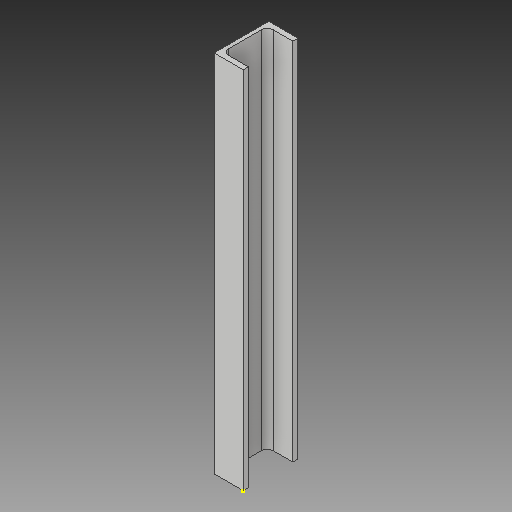
# Autodesk Inventor part: Channel2_CPY
Saved by Autodesk Inventor 2019 (Build 230136000, 136)
## iProperties
Created: 2019-05-26
Part Number: Channel2_CPY
Material: Generic
Document SubType Name: Modeling
Designer: Satwik Pandey
Density: 1 g/cm^3
Appearance: Default
Author: dell
Autodesk Inventor part; units mm, degrees
ref_plane "YZ Plane" through (0, 0, 0) normal (1, 0, 0) x (0, 1, 0)
ref_plane "XZ Plane" through (0, 0, 0) normal (0, 1, 0) x (-1, 0, 0)
ref_plane "XY Plane" through (0, 0, 0) normal (0, 0, 1) x (1, 0, 0)
sketch "Sketch1" plane through (0, 0, 0) normal (0, 1, 0) x (-1, 0, 0)
  point P0 (0, 0)
sketch "Sketch2" plane through (0, 0, 0) normal (0, 1, 0) x (-1, 0, 0)
  line L0 (0, 0) -> (40, 0)
  line L1 (40, 0) -> (40, -75)
  line L2 (40, -75) -> (0, -75)
  line L3 (0, -75) -> (0, -68)
  line L4 (0, -68) -> (27, -68)
  line L5 (35, -60) -> (35, -15)
  line L6 (27, -7) -> (0, -7)
  line L7 (0, -7) -> (0, 0)
  arc A0 (35, -15) -> (27, -7) centre (27, -15) ccw
  arc A1 (27, -68) -> (35, -60) centre (27, -60) ccw
  point P0 (35, -68)
  point P1 (35, -7)
  dimension "d0" = 40
  dimension "d1" = 75
  dimension "d2" = 40
  dimension "d3" = 7
  dimension "d5" = 35
  dimension "d6" = 61
  dimension "d7" = 8
  constraints: 16 end point, 6 perpendicular, 4 point on circle, 4 point on line, 4 tangent, 2 centre point, 2 horizontal, 1 equal radius
  measures "d0" distance of L0.start L0.end
  measures "d1" distance of L0.end L1.end
  measures "d2" distance of L1.end L2.end
  measures "d3" distance of L2.end L3.end
  measures "d5" distance of L3.end point (35, -68)
  measures "d6" distance of point (35, -68) point (35, -7)
  measures "d7" radius of A0
extrude "Extrusion1" add sketch "Sketch2" along normal blind 500
body "Solid1"
